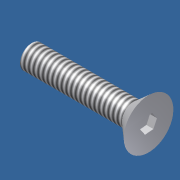
# Autodesk Inventor part: HW-00013
Saved by Autodesk Inventor 2012 (Build 160160000, 160)
## iProperties
Created: 2008-05-28
Part Number: HW-00013
Document SubType Name: Modeling
Designer: mcyr
Density: 1 g/cm^3
Mass: 1.17962 g
Surface Area: 9.21662 cm^2
Volume: 1.17962 cm^3
Description: 1/4-20 x 1-1/4" Flat head screw, zinc plated
Material: Default
Title: HW-00007
Author: mcyr
Autodesk Inventor part; units mm, degrees
ref_plane "YZ Plane" through (0, 0, 0) normal (1, 0, 0) x (0, 1, 0)
ref_plane "XZ Plane" through (0, 0, 0) normal (0, 1, 0) x (-1, 0, 0)
ref_plane "XY Plane" through (0, 0, 0) normal (0, 0, 1) x (1, 0, 0)
sketch "Sketch1" plane through (0, 0, 0) normal (0, 0, 1) x (1, 0, 0)
  line L0 (25.3049, 0.2033) -> (-6.4451, 0.2033)
  line L1 (-6.4451, 0.2033) -> (-6.4451, 3.3783)
  line L2 (-6.4451, 3.3783) -> (21.2155, 3.3783)
  line L3 (21.2155, 3.3783) -> (25.3049, 6.947)
  line L4 (25.3049, 6.947) -> (25.3049, 0.2033)
  dimension "d1" = 3.175
  dimension "d2" = 4.0894
  dimension "d3" = 6.7437
  dimension "d20" = 31.75
  constraints: 10 end point, 2 parallel, 1 horizontal, 1 perpendicular
  measures "d1" distance of L0.end L1.end
  measures "d2" horizontal distance of L3.end L2.end
  measures "d3" distance of L3.end L0.start
  measures "d20" distance of L0.start L0.end
revolve "Revolution1" add sketch "Sketch1" angle 360 about axis through (25.3049, 0.2033, 0) along (-1, 0, 0)
thread "Thread1" size "1/4-20 UNC" class "2A" standard "ANSI Unified Screw Threads" full length
sketch "Sketch2" plane through (25.3049, 0.2033, 0) normal (1, 0, 0) x (0, 0, -1)
  circle A0 centre (0, 0) radius 6.7437 projected
  line L0 (-1.3229, 1.8709) -> (0.9588, 2.0811)
  line L1 (0.9588, 2.0811) -> (2.2817, 0.2103)
  line L2 (2.2817, 0.2103) -> (1.3229, -1.8709)
  line L3 (1.3229, -1.8709) -> (-0.9588, -2.0811)
  line L4 (-0.9588, -2.0811) -> (-2.2817, -0.2103)
  line L5 (-2.2817, -0.2103) -> (-1.3229, 1.8709)
  dimension "d16" = 3.9688
  constraints: 12 end point, 1 coincident, 13 other
  measures "d16" distance between parallel lines of L2 L5
extrude "Extrusion1" cut sketch "Sketch2" against normal blind 1.905 contours L0 L1 L2 L3 L4 L5
body "Solid1"
